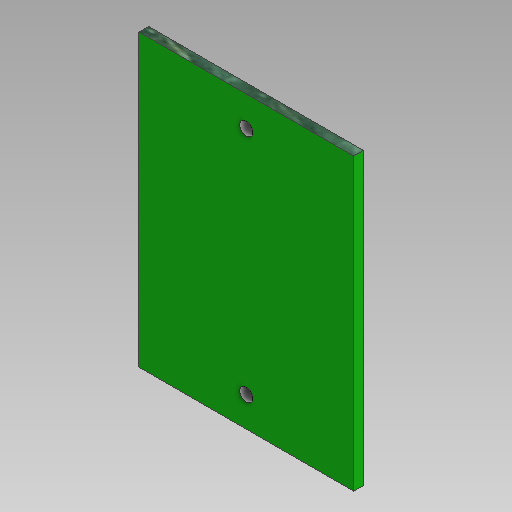
# Autodesk Inventor part: RedLEDArray
Saved by Autodesk Inventor 2026.1 (Build 301233000, 233)
## iProperties
Created: 2026-03-01
Part Number: RedLEDArray
Material: Generic
Document SubType Name: Modeling
Designer: aleja
Density: 1 g/cm^3
Appearance: Default
Author: aleja
Autodesk Inventor part; units mm, degrees
ref_plane "YZ Plane" through (0, 0, 0) normal (1, 0, 0) x (0, 1, 0)
ref_plane "XZ Plane" through (0, 0, 0) normal (0, 1, 0) x (-1, 0, 0)
ref_plane "XY Plane" through (0, 0, 0) normal (0, 0, 1) x (1, 0, 0)
sketch "Sketch1" plane through (0, 0, 0) normal (0, 1, 0) x (-1, 0, 0)
  line L0 (17.75, 24) -> (-17.75, 24)
  line L1 (-17.75, 24) -> (-17.75, -24)
  line L2 (-17.75, -24) -> (17.75, -24)
  line L3 (17.75, -24) -> (17.75, 24)
  line L4 (17.75, 24) -> (-17.75, -24) construction
  line L5 (-17.75, 24) -> (17.75, -24) construction
  point P0 (0, 0)
  dimension "d0" = 35.5
  dimension "d1" = 48
  constraints: 12 end point, 2 midpoint, 2 parallel, 1 horizontal, 1 perpendicular
  measures "d0" distance of L2.end L1.end
  measures "d1" distance of L1.end L0.end
extrude "Extrusion1" add sketch "Sketch1" along normal blind 1.6
sketch "Sketch2" plane through (0, 1.6, 0) normal (0, 1, 0) x (1, 0, 0)
  line L0 (-12, 19.5) -> (-8, 19.5)
  line L1 (-8, 19.5) -> (-8, 15.5)
  line L2 (-8, 15.5) -> (-12, 15.5)
  line L3 (-12, 15.5) -> (-12, 19.5)
  line L4 (-12, 19.5) -> (-8, 15.5) construction
  line L5 (-8, 19.5) -> (-12, 15.5) construction
  line L6 (-17.75, -24) -> (17.75, -24) projected
  line L7 (17.75, 24) -> (-17.75, 24) projected
  line L8 (-17.75, 24) -> (-17.75, -24) projected
  line L9 (17.75, -24) -> (17.75, 24) projected
  line L10 (12, 15.5) -> (8, 15.5)
  line L11 (12, 19.5) -> (12, 15.5)
  line L12 (8, 19.5) -> (12, 19.5)
  line L13 (8, 15.5) -> (8, 19.5)
  line L14 (-8, 8.5) -> (-12, 8.5)
  line L15 (-8, 12.5) -> (-8, 8.5)
  line L16 (-12, 12.5) -> (-8, 12.5)
  line L17 (-12, 8.5) -> (-12, 12.5)
  line L18 (12, 8.5) -> (8, 8.5)
  line L19 (12, 12.5) -> (12, 8.5)
  line L20 (8, 12.5) -> (12, 12.5)
  line L21 (8, 8.5) -> (8, 12.5)
  line L22 (-8, 1.5) -> (-12, 1.5)
  line L23 (-8, 5.5) -> (-8, 1.5)
  line L24 (-12, 5.5) -> (-8, 5.5)
  line L25 (-12, 1.5) -> (-12, 5.5)
  line L26 (12, 1.5) -> (8, 1.5)
  line L27 (12, 5.5) -> (12, 1.5)
  line L28 (8, 5.5) -> (12, 5.5)
  line L29 (8, 1.5) -> (8, 5.5)
  line L30 (-8, -5.5) -> (-12, -5.5)
  line L31 (-8, -1.5) -> (-8, -5.5)
  line L32 (-12, -1.5) -> (-8, -1.5)
  line L33 (-12, -5.5) -> (-12, -1.5)
  line L34 (12, -5.5) -> (8, -5.5)
  line L35 (12, -1.5) -> (12, -5.5)
  line L36 (8, -1.5) -> (12, -1.5)
  line L37 (8, -5.5) -> (8, -1.5)
  line L38 (-8, -12.5) -> (-12, -12.5)
  line L39 (-8, -8.5) -> (-8, -12.5)
  line L40 (-12, -8.5) -> (-8, -8.5)
  line L41 (-12, -12.5) -> (-12, -8.5)
  line L42 (12, -12.5) -> (8, -12.5)
  line L43 (12, -8.5) -> (12, -12.5)
  line L44 (8, -8.5) -> (12, -8.5)
  line L45 (8, -12.5) -> (8, -8.5)
  line L46 (-8, -19.5) -> (-12, -19.5)
  line L47 (-8, -15.5) -> (-8, -19.5)
  line L48 (-12, -15.5) -> (-8, -15.5)
  line L49 (-12, -19.5) -> (-12, -15.5)
  line L50 (12, -19.5) -> (8, -19.5)
  line L51 (12, -15.5) -> (12, -19.5)
  line L52 (8, -15.5) -> (12, -15.5)
  line L53 (8, -19.5) -> (8, -15.5)
  point P0 (0, 0)
  point P1 (-10, 17.5)
  dimension "d4" = 4
  dimension "d5" = 4
  dimension "d6" = 48
  dimension "d7" = 35.5
  dimension "d8" = 17.5
  dimension "d9" = 10
  dimension "d20" = 20
  dimension "d23" = 7
  constraints: 100 end point, 2 collinear, 2 horizontal, 2 midpoint, 2 parallel, 1 perpendicular, 1 vertical, 86 other
  measures "d4" distance of L1.end L2.end
  measures "d5" distance of L0.end L1.end
  measures "d6" distance between parallel lines of L6 L7
  measures "d7" distance between parallel lines of L8 L9
  measures "d8" vertical distance of point (-10, 17.5) point (0, 0)
  measures "d9" horizontal distance of point (0, 0) point (-10, 17.5)
  measures "d20" distance of L1.end L10.start
  measures "d23" distance of L1.end L14.start
extrude "Extrusion2" add sketch "Sketch2" along normal blind 1.6 contours L0 L1 L2 L3 | L10 L13 L12 L11 | L14 L17 L16 L15 | L18 L21 L20 L19 | L22 L25 L24 L23 | L26 L29 L28 L27 | L30 L33 L32 L31 | L34 L37 L36 L35 | L38 L41 L40 L39 | L42 L45 L44 L43 | L46 L49 L48 L47 | L50 L53 L52 L51
sketch "Sketch3" plane through (0, 1.6, 0) normal (0, 1, 0) x (1, 0, 0)
  line L0 (0, 0) -> (0, 19.05) construction
  line L1 (0, 0) -> (4.4844, 0) construction
  circle A0 centre (0, 19.05) radius 1.1
  circle A1 centre (0, -19.05) radius 1.1
  dimension "d28" = 19.05
  dimension "d29" = 2.2
  constraints: 4 end point, 2 centre point, 1 coincident, 1 horizontal, 1 symmetric about line, 1 vertical, 1 other
  measures "d28" distance of L0.start L0.end
  measures "d29" diameter of A0
extrude "Extrusion3" cut sketch "Sketch3" against normal through all
body "Solid1"
